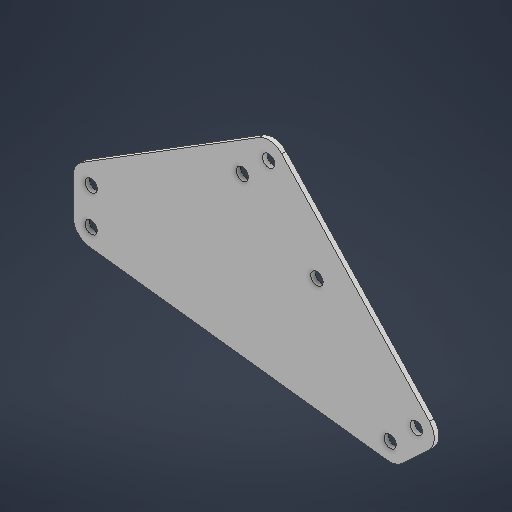
# Autodesk Inventor part: 2.1-Gearbox
Saved by Autodesk Inventor 2026.1 (Build 301233000, 233)
## iProperties
Created: 2025-08-08
Part Number: 2.1-Gearbox
Material: Generic
Document SubType Name: Modeling
Designer: roejo
Density: 1 g/cm^3
Appearance: Default
Author: roejo
Autodesk Inventor part; units mm, degrees
ref_plane "YZ Plane" through (0, 0, 0) normal (1, 0, 0) x (0, 1, 0)
ref_plane "XZ Plane" through (0, 0, 0) normal (0, 1, 0) x (-1, 0, 0)
ref_plane "XY Plane" through (0, 0, 0) normal (0, 0, 1) x (1, 0, 0)
sketch "Sketch1" plane through (0, 0, 0) normal (0, 0, 1) x (1, 0, 0)
  circle A0 centre (48.2493, -30.8623) radius 2.1844
  circle A1 centre (57.5164, -22.1784) radius 2.1844
  circle A2 centre (5.4131, 33.4246) radius 2.1844
  circle A3 centre (-3.854, 24.7407) radius 2.1844
  circle A4 centre (22.4893, 5.9147) radius 2.1844
  circle A5 centre (-57.1544, -5.4775) radius 2.1844 construction
  circle A6 centre (-57.1544, -18.1775) radius 2.1844 construction
  arc A7 (-60.5073, -0.0848) -> (-63.5044, -5.4775) centre (-57.1544, -5.4775) ccw
  arc A8 (-63.5044, -18.1775) -> (-57.9131, -24.482) centre (-57.1544, -18.1775) ccw
  circle A9 centre (-57.1544, -5.4775) radius 2.1844
  circle A10 centre (-57.1544, -18.1775) radius 2.1844
  arc A11 (10.0467, 37.7665) -> (2.0602, 38.8172) centre (5.4131, 33.4246) ccw
  arc A12 (61.8584, -26.812) -> (62.15, -17.8364) centre (57.5164, -22.1784) ccw
  arc A13 (47.4906, -37.1668) -> (52.5912, -35.4958) centre (48.2493, -30.8623) ccw
  line L0 (10.0467, 37.7665) -> (62.15, -17.8364)
  line L1 (61.8584, -26.812) -> (52.5912, -35.4958)
  line L2 (47.4906, -37.1668) -> (-57.9131, -24.482)
  line L3 (-63.5044, -18.1775) -> (-63.5044, -5.4775)
  line L4 (-60.5073, -0.0848) -> (2.0602, 38.8172)
  dimension "d0" = 12.7
  dimension "d1" = 12.7
  dimension "d2" = 12.7
  dimension "d3" = 12.7
  dimension "d4" = 12.7
  constraints: 14 centre point, 10 end point, 10 point on circle, 9 tangent, 7 coincident, 2 concentric, 1 perpendicular, 5 other
  measures "d0" diameter of A7
  measures "d1" diameter of A8
  measures "d2" diameter of A11
  measures "d3" diameter of A12
  measures "d4" diameter of A13
extrude "Extrusion1" add sketch "Sketch1" along normal blind 1.5875
body "Solid1"
